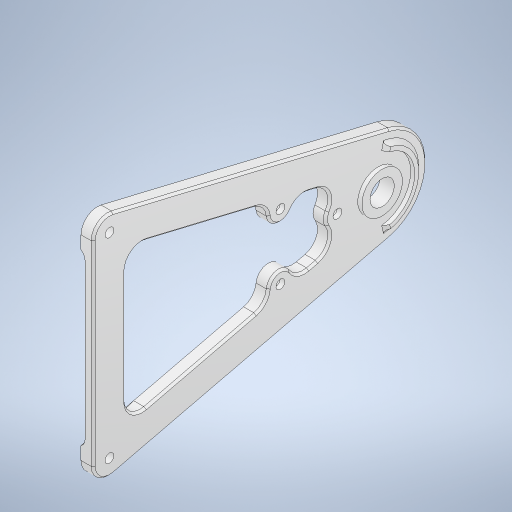
# Autodesk Inventor part: Upright - Blank
Saved by Autodesk Inventor 2023.2 (Build 272271000, 271)
## iProperties
Created: 2023-07-17
Part Number: Upright - Blank
Material: Aluminum 6061
Document SubType Name: Modeling
Designer: Nathan Cai
Mass: 56.1067 g
Surface Area: 124.558 cm^2
Volume: 20.7802 cm^3
Density: 2.7 g/cm^3
Appearance: Aluminum - Flat
Author: Nathan Cai
Autodesk Inventor part; units mm, degrees
ref_plane "YZ Plane" through (0, 0, 0) normal (1, 0, 0) x (0, 1, 0)
ref_plane "XZ Plane" through (0, 0, 0) normal (0, 1, 0) x (-1, 0, 0)
ref_plane "XY Plane" through (0, 0, 0) normal (0, 0, 1) x (1, 0, 0)
sketch "Sketch1" plane through (0, 0, 0) normal (1, 0, 0) x (0, 1, 0)
  circle A0 centre (0, 0) radius 3.5 construction
  circle A1 centre (38.1, -6.35) radius 1.7526
  circle A2 centre (38.1, -6.35) radius 6.35
  line L0 (0, 0) -> (0, -111.125) construction
  circle A3 centre (0, -111.125) radius 4.7625
  circle A4 centre (0, -111.125) radius 19.05
  circle A5 centre (0, -95.25) radius 1.7526
  circle A6 centre (0, -95.25) radius 4.7625
  line L1 (44.276, -7.8261) -> (18.5281, -115.5534)
  line L2 (31.924, -4.8739) -> (10.3512, -95.1326)
  circle A7 centre (12.7, -73.025) radius 1.7526
  circle A8 centre (12.7, -73.025) radius 4.7625
  circle A9 centre (-38.1, -6.35) radius 1.7526
  circle A10 centre (-38.1, -6.35) radius 6.35
  line L3 (-44.276, -7.8261) -> (-18.5281, -115.5534)
  line L4 (-31.924, -4.8739) -> (-10.3512, -95.1326)
  circle A11 centre (-12.7, -73.025) radius 1.7526
  circle A12 centre (-12.7, -73.025) radius 4.7625
  line L5 (-38.1, 0) -> (38.1, 0)
  line L6 (38.1, -12.7) -> (-38.1, -12.7)
  point P0 (39.9083, -0.2629)
  point P1 (-39.9083, -0.2629)
  point P2 (16.3627, -69.981)
  point P3 (14.5904, -77.3963)
  point P4 (3.8683, -92.4719)
  point P5 (-3.8683, -92.4719)
  point P6 (-14.5904, -77.3963)
  point P7 (-16.3627, -69.981)
  point P8 (-30.0534, -12.7)
  point P9 (30.0534, -12.7)
  dimension "d0" = 7
  dimension "d2" = 3.5052
  dimension "d3" = 12.7
  dimension "d4" = 38.1
  dimension "d5" = 6.35
  dimension "d6" = 111.125
  dimension "d7" = 9.525
  dimension "d8" = 38.1
  dimension "d9" = 3.5052
  dimension "d10" = 9.525
  dimension "d11" = 15.875
  dimension "d12" = 12.7
  dimension "d13" = 3.5052
  dimension "d14" = 9.525
  dimension "d15" = 12.7
  dimension "d16" = 38.1
  constraints: 14 end point, 13 centre point, 12 point on circle, 9 coincident, 9 symmetric about line, 6 tangent, 1 parallel, 1 point on line, 1 vertical, 4 other
  measures "d0" diameter of A0
  measures "d2" diameter of A1
  measures "d3" diameter of A2
  measures "d4" horizontal distance of L0.start A1.centre
  measures "d5" vertical distance of L0.start A1.centre
  measures "d6" distance of L0.start L0.end
  measures "d7" diameter of A3
  measures "d8" diameter of A4
  measures "d9" diameter of A5
  measures "d10" diameter of A6
  measures "d11" distance of A3.centre A6.centre
  measures "d12" distance between parallel lines of L1 L2
  measures "d13" diameter of A7
  measures "d14" diameter of A8
  measures "d15" distance from line of L0 A8.centre
  measures "d16" vertical distance of A3.centre A8.centre
extrude "Extrusion1" add sketch "Sketch1" along normal blind 4.7625 contours A2 | A2 L2 L6 L4 A10 L5 | L1 A4 L2 A8 L6 A2 | A2 L6 L2 | A10 | A4 A6 | L4 L6 A10 | A10 L6 L4 A12 A4 L3 | A8 L2 | L2 A8 | A12 L4 | L4 A12 | A6 A4 | A4 A6
fillet "Fillet1" radius 6.35 10 edges at (2.3813, 16.3627, -69.981) (2.3813, 14.5904, -77.3963) (2.3813, 3.8683, -92.4719) (2.3813, -3.8683, -92.4719) (2.3813, -14.5904, -77.3963) (2.3813, -16.3627, -69.981) (2.3813, 10.3512, -95.1326) (2.3813, -10.3512, -95.1326) (2.3813, -30.0534, -12.7) (2.3813, 30.0534, -12.7)
sketch "Sketch2" plane through (4.7625, 0, 0) normal (1, 0, 0) x (0, 0, -1)
  circle A0 centre (111.125, 0) radius 4.7625 projected
  circle A1 centre (111.125, 0) radius 14.2875
  circle A2 centre (111.125, 0) radius 12.7
  arc A3 (115.5534, -18.5281) -> (115.5534, 18.5281) centre (111.125, 0) ccw projected
  line L0 (111.125, 0) -> (115.5534, -18.5281)
  line L1 (115.5534, 18.5281) -> (7.8261, 44.276) projected
  line L2 (111.125, 0) -> (115.5534, 18.5281)
  point P0 (0, 0)
  point P1 (114.4463, 13.8961)
  point P2 (114.0773, 12.3521)
  point P3 (114.0773, -12.3521)
  point P4 (114.4463, -13.8961)
  point P5 (92.4719, -3.8683)
  point P6 (92.4719, 3.8683)
  dimension "d20" = 28.575
  dimension "d21" = 1.5875
  constraints: 4 end point, 2 centre point, 1 coincident, 1 perpendicular
  measures "d20" diameter of A1
  measures "d21" radial gap between concentric circles of A1 A2
extrude "Extrusion2" add sketch "Sketch2" along normal blind 1.5875 contours L2 A1 L0 A2 picked at (124.6612, 1.9868)
fillet "Fillet2" radius 1.5875 1 edges at (4.7625, 0, -125.4125)
chamfer "Chamfer1" distance 1.5875 angle 45 4 edges at (4.7625, -14.6681, -114.6308) (4.7625, -13.1241, -114.2618) (4.7625, 14.6681, -114.6308) (4.7625, 13.1241, -114.2618)
sketch "Sketch3" plane through (0, 0, 0) normal (-1, 0, 0) x (0, 0, 1)
  circle A0 centre (-111.125, 0) radius 4.7625 projected
  circle A1 centre (-111.125, 0) radius 11.1125
  arc A2 (-7.8261, -44.276) -> (0, -38.1) centre (-6.35, -38.1) ccw projected
  line L0 (0, 38.1) -> (0, -38.1) projected
  arc A3 (0, 38.1) -> (-7.8261, 44.276) centre (-6.35, 38.1) ccw projected
  line L1 (-115.5534, 18.5281) -> (-7.8261, 44.276) projected
  arc A4 (-115.5534, 18.5281) -> (-115.5534, -18.5281) centre (-111.125, 0) ccw projected
  line L2 (-7.8261, -44.276) -> (-115.5534, -18.5281) projected
  circle A5 centre (-6.35, -38.1) radius 1.7526 projected
  circle A6 centre (-95.25, 0) radius 1.7526 projected
  circle A7 centre (-73.025, 12.7) radius 1.7526 projected
  arc A8 (-87.3893, 12.2019) -> (-91.2485, 2.5825) centre (-85.9132, 6.0259) ccw projected
  line L3 (-83.9481, 13.0244) -> (-87.3893, 12.2019) projected
  arc A9 (-77.0737, 10.1922) -> (-83.9481, 13.0244) centre (-82.472, 6.8484) ccw projected
  arc A10 (-77.0737, 10.1922) -> (-68.2798, 12.294) centre (-73.025, 12.7) ccw projected
  arc A11 (-63.4291, 17.9287) -> (-68.2798, 12.294) centre (-61.953, 11.7526) ccw projected
  line L4 (-20.5261, 28.1829) -> (-63.4291, 17.9287) projected
  arc A12 (-12.7, 22.0069) -> (-20.5261, 28.1829) centre (-19.05, 22.0069) ccw projected
  line L5 (-12.7, -22.0069) -> (-12.7, 22.0069) projected
  arc A13 (-20.5261, -28.1829) -> (-12.7, -22.0069) centre (-19.05, -22.0069) ccw projected
  line L6 (-63.4291, -17.9287) -> (-20.5261, -28.1829) projected
  arc A14 (-68.2798, -12.294) -> (-63.4291, -17.9287) centre (-61.953, -11.7526) ccw projected
  arc A15 (-68.2798, -12.294) -> (-77.0737, -10.1922) centre (-73.025, -12.7) ccw projected
  arc A16 (-83.9481, -13.0244) -> (-77.0737, -10.1922) centre (-82.472, -6.8484) ccw projected
  line L7 (-87.3893, -12.2019) -> (-83.9481, -13.0244) projected
  arc A17 (-91.2485, -2.5825) -> (-87.3893, -12.2019) centre (-85.9132, -6.0259) ccw projected
  arc A18 (-91.2485, -2.5825) -> (-91.2485, 2.5825) centre (-95.25, 0) ccw projected
  circle A19 centre (-73.025, -12.7) radius 1.7526 projected
  circle A20 centre (-111.125, 0) radius 4.7625 projected
  circle A21 centre (-6.35, 38.1) radius 1.7526 projected
  line L8 (-20.5261, 28.1829) -> (0, 33.0889)
  line L9 (0, 38.1) -> (0, -38.1) projected
  line L10 (-20.5261, 28.1829) -> (-63.4291, 17.9287) projected
  line L11 (-95.25, 0) -> (0, 0) construction
  line L12 (-12.7, -22.0069) -> (-12.7, 22.0069) projected
  line L13 (-20.5261, -28.1829) -> (0, -33.0889)
  point P0 (0, -33.0889)
  point P1 (0, 33.0889)
  dimension "d31" = 22.225
  constraints: 6 end point, 1 centre point, 1 coincident, 1 collinear, 1 perpendicular, 1 point on line, 1 symmetric about line
  measures "d31" diameter of A1
extrude "Extrusion3" cut sketch "Sketch3" against normal blind 0.7937 contours A0 | A1
extrude "Extrusion4" cut sketch "Sketch3" against normal blind 1.5875 contours L13 A13 L5 A12 L8 L0
fillet "Fillet3" radius 3.175 2 edges at (1.5875, 30.6359, -10.2631) (1.5875, -30.6359, -10.2631)
sketch "Sketch4" plane through (4.7625, 0, 0) normal (1, 0, 0) x (0, 0, -1)
  circle A0 centre (111.125, 0) radius 4.7625 projected
  circle A1 centre (111.125, 0) radius 7.9375
  point P0 (0, 0)
  dimension "d38" = 15.875
  constraints: 1 centre point, 1 coincident
  measures "d38" diameter of A1
extrude "Extrusion5" add sketch "Sketch4" along normal blind 1.5875
chamfer "Chamfer2" distance 0.7937 angle 45 23 edges at (4.7625, -31.4021, -61.6898) (4.7625, 0, -130.175) (4.7625, 31.4021, -61.6898) (4.7625, 43.0848, -2.4162) (4.7625, -28.7762, 0) (4.7625, 9.3238, 0) (4.7625, -43.0848, -2.4162) (4.7625, -12.7196, -80.0531) (4.7625, -12.613, -85.6694) (4.7625, -8.3902, -91.8074) (4.7625, 0, -90.4875) (4.7625, 8.3901, -91.8074) (4.7625, 12.613, -85.6694) (4.7625, 12.7196, -80.0531) (4.7625, 8.068, -71.9179) (4.7625, 15.8955, -66.7654) (4.7625, 23.0558, -41.9776) (4.7625, 26.9916, -15.1162) (4.7625, 0, -12.7) (4.7625, -26.9916, -15.1162) (4.7625, -23.0558, -41.9776) (4.7625, -15.8955, -66.7654) (4.7625, -8.068, -71.9179)
chamfer "Chamfer3" distance 2.54 angle 49 3 edges at (0, -14.4526, -73.025) (0, 10.9474, -73.025) (0, -1.7526, -95.25) measured on face at (0, 10.4474, -73.025) measured on face at (0, -14.9526, -73.025) measured on face at (0, -2.2526, -95.25)
equation "\"d4\" = S_Offset"
equation "\"d5\" = M2S"
equation "\"d6\" = C2C"
equation "\"d7\" = Bore"
equation "\"d8\" = FrontOD"
equation "\"d11\" = Leg_X_Front"
equation "\"d15\" = Leg_Y_Back"
equation "\"d16\" = Leg_X_Back"
equation "\"S_Offset\" = 38.1"
equation "\"M2S\" = 6.35"
equation "\"C2C\" = 111.125"
equation "\"Bore\" = 9.525"
equation "\"FrontOD\" = 38.1"
equation "\"Leg_X_Front\" = 15.875"
equation "\"Leg_Y_Back\" = 12.7"
equation "\"Leg_X_Back\" = 38.1"
body "Solid1"
